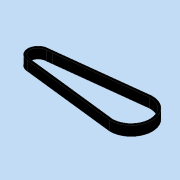
# Autodesk Inventor part: Pas zębaty 10 T5-295
Saved by Autodesk Inventor 2018 (Build 220112000, 112)
## iProperties
Created: 2019-01-29
Part Number: Pas zębaty 10 T5-295
Material: Ogólny
Document SubType Name: Modeling
Designer: Dawid
Density: 1 g/cm^3
Appearance: Anodowana - czarna
Author: Dawid
Autodesk Inventor part; units mm, degrees
ref_plane "YZ Plane" through (0, 0, 0) normal (1, 0, 0) x (0, 1, 0)
ref_plane "XZ Plane" through (0, 0, 0) normal (0, 1, 0) x (-1, 0, 0)
ref_plane "XY Plane" through (0, 0, 0) normal (0, 0, 1) x (1, 0, 0)
sketch "Szkic1" plane through (0, 0, 0) normal (0, 0, 1) x (1, 0, 0)
  line L0 (0, 0) -> (-96.26, 0)
  circle A0 centre (0, 0) radius 15
  circle A1 centre (-96.26, 0) radius 4
  line L1 (-96.26, 10.725) -> (0, 21.875)
  line L2 (0, -21.875) -> (-96.26, -10.725)
  line L3 (-51.7735, 15.878) -> (-40.2853, 17.2087) construction
  line L4 (-51.7735, 15.878) -> (-40.2853, 17.2087) construction
  line L5 (-96.26, 10.725) -> (-84.9982, 12.0295) construction
  line L6 (-90.2773, 8.9013) -> (-51.4859, 13.3946)
  line L7 (0, 21.875) -> (-10.2296, 20.6901) construction
  line L8 (-12.5709, 17.9022) -> (-51.4859, 13.3946)
  arc A2 (-92.5853, 0) -> (-92.2617, 0.1164) centre (-96.26, 10.725) ccw
  line L9 (-96.26, -10.725) -> (-94.0957, -10.9757) construction
  line L10 (0, -21.875) -> (-6.8977, -21.076) construction
  line L11 (-12.5709, -17.9022) -> (-90.2773, -8.9013)
  line L12 (0.7988, -14.9787) -> (0.799, -14.9773) construction
  line L13 (0.799, -14.9773) -> (0.7988, -14.9787)
  arc A3 (-12.5709, 17.9022) -> (-12.5709, -17.9022) centre (0, 0) ccw
  arc A4 (0, -21.875) -> (0, 21.875) centre (0, 0) ccw
  line L14 (-96.26, 0) -> (-96.26, 8.225)
  circle A5 centre (-96.26, 0) radius 8.225
  line L15 (-90.2773, -8.9013) -> (-96.26, -8.225)
  arc A6 (-96.26, 10.725) -> (-96.26, -10.725) centre (-96.26, 0) ccw
  arc A7 (-90.2773, -8.9013) -> (-90.2773, 8.9013) centre (-96.26, 0) ccw
  line L16 (0.0019, -0.0165) -> (0.0019, 19.3585)
  circle A8 centre (0.0019, -0.0165) radius 19.375
  line L17 (-12.5709, 17.9022) -> (0.0019, 19.3585)
  line L18 (-12.5709, -17.9022) -> (0.0019, -19.3915)
  line L19 (-96.26, 8.225) -> (-90.2773, 8.9013)
  dimension "d0" = 96.26
  dimension "d16" = 19.375
  dimension "d17" = 8.225
  constraints: 40 end point, 16 point on circle, 7 centre point, 7 point on line, 5 coincident, 2 collinear, 2 vertical, 1 horizontal, 6 other
  measures "d0" distance of L0.start L0.end
  measures "d16" distance of L16.start L16.end
  measures "d17" distance of L14.start L14.end
extrude "Wyciągnięcie proste1" add sketch "Szkic1" along normal blind 10 contours A8 L17 | L18 A8 | L1 A4 L2 A6
